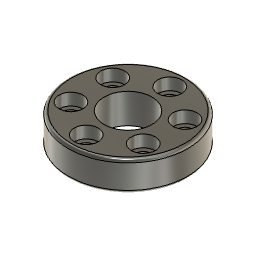
WheelHub (Autodesk Fusion 360 design; units mm, degrees)
Autodesk Fusion 360 part; units mm, degrees
sketch "Sketch1" plane through (0, 0, 0) normal (0, 0, 1) x (1, 0, 0)
  circle A0 centre (0, 0) radius 12.7
  circle A1 centre (0, 0) radius 5.08
  dimension "d1" = 25.4
  dimension "d3" = 10.16
  constraint coincident A0.centre A1.centre
  constraint concentric A0 A1
  measures "d1" diameter of A0
  measures "d3" diameter of A1
extrude "Extrude1" add sketch "Sketch1" along normal blind 6.35
sketch "Sketch3" plane through (0, 0, 6.35) normal (0, 0, 1) x (-1, 0, 0)
  circle A0 centre (0, 0) radius 5.08
  circle A1 centre (0, 0) radius 12.7
  line L0 (0, 5.08) -> (0, 12.7)
  circle A2 centre (0, 0) radius 8.89
  point P0 (0, 8.89)
  constraint coincident A1 L0.end
  constraint vertical L0
  constraint coincident A0.centre A1.centre
  constraint vertical L0.end A0.centre
  constraint midpoint L0 P0
  constraint coincident A2 P0
  constraint coincident A0 L0.start
hole "Hole1" at (0, -8.89, 6.35) direction (0, 0, -1) diameter 3.175 depth 6.35 tip angle 180 counterbore diameter 5.08 counterbore depth 2.54
pattern_circular "C-Pattern1" count 6 over 360 about axis through (0, 0, 0) along (0, 0, 1) of "Hole1"
fillet "Fillet1" radius 0.635 2 edges at (-11.8406, -4.5925, 6.35) (-11.8406, -4.5925, 0)
